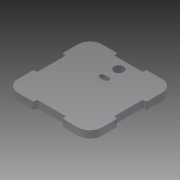
# Autodesk Inventor part: 020914 Aft Outer Endcap
Saved by Autodesk Inventor 2015 (Build 190159000, 159)
## iProperties
Created: 2013-05-23
Part Number: 020914 Aft Outer Endcap
Material: Polycarbonate, Clear
Document SubType Name: Modeling
Designer: Eric
Density: 1.2 g/cm^3
Mass: 2.90508 g
Surface Area: 20.2664 cm^2
Volume: 2.4209 cm^3
Appearance: Polycarbonate - Clear
Author: Eric
Autodesk Inventor part; units mm, degrees
ref_plane "YZ Plane" through (0, 0, 0) normal (1, 0, 0) x (0, 1, 0)
ref_plane "XZ Plane" through (0, 0, 0) normal (0, 1, 0) x (-1, 0, 0)
ref_plane "XY Plane" through (0, 0, 0) normal (0, 0, 1) x (1, 0, 0)
sketch "Sketch1" plane through (0, 0, 0) normal (0, 0, 1) x (1, 0, 0)
  circle A0 centre (0, 12) radius 2
  line L0 (-17, -6) -> (-16.5, -6)
  line L1 (-16, -5.5) -> (-16, 5.5)
  line L2 (-16.5, 6) -> (-17, 6)
  line L3 (-17.5, 12.5) -> (-17.5, 6.5)
  line L4 (-17.5, -6.5) -> (-17.5, -12.5)
  arc A1 (-16.5, -6) -> (-16, -5.5) centre (-16.5, -5.5) ccw
  arc A2 (-16, 5.5) -> (-16.5, 6) centre (-16.5, 5.5) ccw
  arc A3 (-17.5, 6.5) -> (-17, 6) centre (-17, 6.5) ccw
  arc A4 (-17, -6) -> (-17.5, -6.5) centre (-17, -6.5) ccw
  line L5 (6, -17) -> (6, -16.5)
  line L6 (5.5, -16) -> (-5.5, -16)
  line L7 (-6, -16.5) -> (-6, -17)
  arc A5 (6, -16.5) -> (5.5, -16) centre (5.5, -16.5) ccw
  arc A6 (-5.5, -16) -> (-6, -16.5) centre (-5.5, -16.5) ccw
  arc A7 (-6.5, -17.5) -> (-6, -17) centre (-6.5, -17) ccw
  arc A8 (6, -17) -> (6.5, -17.5) centre (6.5, -17) ccw
  line L8 (17, 6) -> (16.5, 6)
  line L9 (16, 5.5) -> (16, -5.5)
  line L10 (16.5, -6) -> (17, -6)
  arc A9 (16.5, 6) -> (16, 5.5) centre (16.5, 5.5) ccw
  arc A10 (16, -5.5) -> (16.5, -6) centre (16.5, -5.5) ccw
  arc A11 (17.5, -6.5) -> (17, -6) centre (17, -6.5) ccw
  arc A12 (17, 6) -> (17.5, 6.5) centre (17, 6.5) ccw
  line L11 (-6, 17) -> (-6, 16.5)
  line L12 (-5.5, 16) -> (5.5, 16)
  line L13 (6, 16.5) -> (6, 17)
  arc A13 (-6, 16.5) -> (-5.5, 16) centre (-5.5, 16.5) ccw
  arc A14 (5.5, 16) -> (6, 16.5) centre (5.5, 16.5) ccw
  arc A15 (6.5, 17.5) -> (6, 17) centre (6.5, 17) ccw
  arc A16 (-6, 17) -> (-6.5, 17.5) centre (-6.5, 17) ccw
  line L14 (12.5, 17.5) -> (6.5, 17.5)
  line L15 (-6.5, 17.5) -> (-12.5, 17.5)
  line L16 (17.5, -12.5) -> (17.5, -6.5)
  line L17 (17.5, 6.5) -> (17.5, 12.5)
  line L18 (-12.5, -17.5) -> (-6.5, -17.5)
  line L19 (6.5, -17.5) -> (12.5, -17.5)
  arc A17 (-17.5, -12.5) -> (-12.5, -17.5) centre (-12.5, -12.5) ccw
  arc A18 (-12.5, 17.5) -> (-17.5, 12.5) centre (-12.5, 12.5) ccw
  arc A19 (17.5, 12.5) -> (12.5, 17.5) centre (12.5, 12.5) ccw
  arc A20 (12.5, -17.5) -> (17.5, -12.5) centre (12.5, -12.5) ccw
  point P0 (0, 0)
  point P1 (16, 0)
  point P2 (-16, 6)
  point P3 (-16, -6)
  point P4 (-16, 0)
  point P5 (-6, -16)
  point P6 (6, -16)
  point P7 (0, -16)
  point P8 (16, -6)
  point P9 (16, 6)
  point P10 (6, 16)
  point P11 (-6, 16)
  point P12 (0, 16)
  dimension "d6" = 4
  dimension "d44" = 12
  dimension "d45" = 0.5
  dimension "d48" = 360
  dimension "d50" = 5
  dimension "d64" = 12
  dimension "d65" = 16
  dimension "d66" = 35
  constraints: 40 end point, 40 point on circle, 21 centre point, 16 point on line, 16 tangent, 9 parallel, 6 equal radius, 5 perpendicular, 3 horizontal, 3 midpoint, 1 horizontal alignment, 1 vertical alignment, 89 other
  measures "d6" diameter of A0
  measures "d44" distance of point (-16, -6) point (-16, 6)
  measures "d45" radius of A1
  measures "d50" radius of A17
  measures "d64" distance of point (0, 0) A0.centre
  measures "d65" distance from line of point (0, 0) L1
  measures "d66" distance between parallel lines of L18 L15
extrude "Extrusion6" add sketch "Sketch1" along normal blind 3
sketch "Sketch4" plane through (0, 0, 3) normal (0, 0, 1) x (1, 0, 0)
  line L0 (-1, 7) -> (1, 7)
  line L1 (2, 6) -> (2, 6)
  line L2 (1, 5) -> (-1, 5)
  line L3 (-2, 6) -> (-2, 6)
  arc A0 (-1, 7) -> (-2, 6) centre (-1, 6) ccw
  arc A1 (2, 6) -> (1, 7) centre (1, 6) ccw
  arc A2 (1, 5) -> (2, 6) centre (1, 6) ccw
  arc A3 (-2, 6) -> (-1, 5) centre (-1, 6) ccw
  point P0 (0, 0)
  point P1 (-2, 7)
  point P2 (2, 5)
  point P3 (-2, 5)
  point P4 (0, 5)
  dimension "d76" = 2
  dimension "d77" = 4
  dimension "d78" = 5
  dimension "d79" = 1
  constraints: 8 end point, 8 point on circle, 8 tangent, 6 point on line, 4 centre point, 2 equal radius, 2 parallel, 1 concentric, 1 horizontal, 1 midpoint, 1 perpendicular, 1 vertical alignment
  measures "d76" distance of point (-2, 5) point (-2, 7)
  measures "d77" distance of point (2, 5) point (-2, 5)
  measures "d78" distance from line of point (0, 0) L2
  measures "d79" radius of A0
extrude "Extrusion8" cut sketch "Sketch4" against normal through all
body "Solid6"
